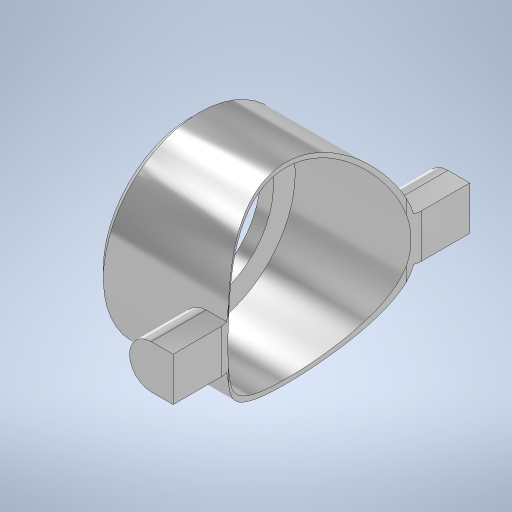
# Autodesk Inventor part: Cup
Saved by Autodesk Inventor 2023.2 (Build 272271000, 271)
## iProperties
Created: 2024-01-10
Part Number: Cup
Material: Aluminum 6061
Document SubType Name: Modeling
Designer: Nathan Cai
Density: 2.7 g/cm^3
Appearance: Aluminum - Flat
Mass: 4.28986 g
Surface Area: 22.2307 cm^2
Volume: 1.58884 cm^3
Author: Nathan Cai
Autodesk Inventor part; units mm, degrees
ref_plane "YZ Plane" through (0, 0, 0) normal (1, 0, 0) x (0, 1, 0)
ref_plane "XZ Plane" through (0, 0, 0) normal (0, 1, 0) x (-1, 0, 0)
ref_plane "XY Plane" through (0, 0, 0) normal (0, 0, 1) x (1, 0, 0)
sketch "Sketch1" plane through (0, 0, 0) normal (1, 0, 0) x (0, 1, 0)
  circle A0 centre (0, 0) radius 11
  circle A1 centre (0, 0) radius 8
  dimension "d0" = 22
  dimension "d3" = 16
  constraints: 2 centre point, 2 coincident
  measures "d0" diameter of A0
  measures "d3" diameter of A1
extrude "Extrusion1" add sketch "Sketch1" along normal blind 15
sketch "Sketch2" plane through (0, 0, 0) normal (0, 0, 1) x (1, 0, 0)
  line L0 (17.5, 2.5) -> (12.5, 2.5)
  line L1 (12.5, 2.5) -> (12.5, -2.5)
  line L2 (12.5, -2.5) -> (17.5, -2.5)
  line L3 (17.5, -2.5) -> (17.5, 2.5)
  line L4 (15, -11) -> (15, 11) projected
  line L5 (17.5, 2.5) -> (12.5, -2.5) construction
  line L6 (12.5, 2.5) -> (17.5, -2.5) construction
  circle A0 centre (12.5, 0) radius 2.5
  point P0 (0, 0)
  point P1 (15, 0)
  point P2 (15, -2.5)
  point P3 (15, 2.5)
  dimension "d4" = 5
  dimension "d5" = 5
  constraints: 12 end point, 4 midpoint, 2 parallel, 1 horizontal, 1 perpendicular, 3 other
  measures "d4" distance of L2.end L1.end
  measures "d5" distance of L1.end L0.end
extrude "Extrusion2" add sketch "Sketch2" along normal mid plane 34 contours L4 A0 L0 | A0 L1 | L1 A0 | L4 L2 A0
sketch "Sketch3" plane through (15, 0, 0) normal (1, 0, 0) x (0, 0, -1)
  circle A0 centre (0, 0) radius 10.5
  dimension "d8" = 21
  constraints: 1 centre point, 1 coincident
  measures "d8" diameter of A0
extrude "Extrusion3" cut sketch "Sketch3" against normal blind 13.5
chamfer "Chamfer1" distance 1 angle 45 1 edges at (0, -11, 0)
sketch "Sketch4" plane through (0, 0, 0) normal (0, 1, 0) x (-1, 0, 0)
  line L0 (-15, 10.7121) -> (-15, -10.7121) projected
  circle A0 centre (-27, 0) radius 16.0857
  line L1 (-15, 0) -> (-27, 0) construction
  point P0 (0, 0)
  dimension "d14" = 12
  constraints: 2 end point, 1 horizontal, 1 midpoint, 3 other
  measures "d14" distance from line of L0 L1.end
extrude "Extrusion4" cut sketch "Sketch4" along normal through all both and the other way through all contours A0 L0 picked at (-13.6381, 0)
fillet "Fillet1" radius 2 2 edges at (15, 0, 10.7121) (15, 0, -10.7121)
body "Solid1"
